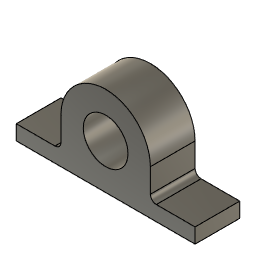
Tutorial Part 3 v1 (Autodesk Fusion 360 design; units mm, degrees)
Autodesk Fusion 360 part; units mm, degrees
sketch "Sketch1" plane through (0, 0, 0) normal (0, 1, 0) x (1, 0, 0)
  line L0 (-60.0453, 0.0038) -> (60.0453, 0.0038)
  line L1 (60.0453, 0.0038) -> (60.0453, -10.0038)
  line L2 (60.0453, -10.0038) -> (-60.0453, -10.0038)
  line L3 (-60.0453, -10.0038) -> (-60.0453, 0.0038)
  line L4 (-60.0453, 0.0038) -> (60.0453, -10.0038) construction
  line L5 (60.0453, 0.0038) -> (-60.0453, -10.0038) construction
  line L6 (-30, -10) -> (30, -10)
  line L7 (30, -10) -> (30, -30)
  line L8 (-30, -30) -> (-30, -10)
  line L9 (-30, -10) -> (30, -30) construction
  line L10 (30, -10) -> (-30, -30) construction
  arc A0 (-30, -30) -> (30, -30) centre (0, -30) ccw
  circle A1 centre (0, -30) radius 15
  line L11 (30, -30) -> (15, -30)
  line L12 (-15, -30) -> (-30, -30)
  point P0 (0, -5)
  point P1 (0, -20)
  dimension "d3" = 60
  dimension "d4" = 20
  constraint horizontal L0
  constraint perpendicular L0 L1
  constraint parallel L1 L3
  constraint coincident L4 P0
  constraint coincident L5 P0
  constraint horizontal L6
  constraint perpendicular L6 L7
  constraint parallel L6 L11
  constraint parallel L7 L8
  constraint coincident L9 P1
  constraint coincident L10 P1
  constraint coincident L8 L10.end
  constraint coincident L10 L8.start
  constraint concentric A0 A1
  constraint coincident A1 L11.end
  constraint coincident A1 L12.start
  constraint collinear L11 L12
  constraint coincident A0.centre L11
  measures "d3" distance of L7.end L8.start
  measures "d4" distance of L6.start L8.start
sketch "Sketch2" plane through (0, 0, 0) normal (0, 1, 0) x (1, 0, 0)
  line L0 (60, 30) -> (-60, 30)
  line L1 (-60, 30) -> (-60, 20)
  line L2 (-60, 20) -> (-30, 20)
  line L3 (-30, 20) -> (-30, 0)
  arc A0 (-30, 0) -> (30, 0) centre (0, 0) ccw
  line L4 (30, 0) -> (30, 20)
  line L5 (30, 20) -> (60, 20)
  line L6 (60, 20) -> (60, 30)
  dimension "d11" = 120
  dimension "d12" = 60
  dimension "d13" = 30
  dimension "d14" = 30
  dimension "d15" = 10
  constraint horizontal L0
  constraint perpendicular L0 L1
  constraint perpendicular L1 L2
  constraint perpendicular L2 L3
  constraint tangent L3 A0
  constraint perpendicular L2 L4
  constraint perpendicular L4 L5
  constraint perpendicular L0 L6
  constraint tangent A0 L4
  constraint coincident A0.centre origin
  constraint collinear L2 L5
  measures "d11" distance of L0.start L0.end
  measures "d12" distance of L1 A0.centre
  measures "d13" radius of A0
  measures "d14" distance of A0.centre L0
  measures "d15" distance of L0.start L5.end
extrude "Extrude2" add sketch "Sketch2" along normal blind 30
sketch "Sketch3" plane through (0, 0, 0) normal (0, -1, 0) x (1, 0, 0)
  line L0 (60, -30) -> (60, -20)
  line L1 (60, -20) -> (30, -20)
  line L2 (30, -20) -> (30, 0)
  arc A0 (30, 0) -> (-30, 0) centre (0, 0) ccw
  line L3 (-30, 0) -> (-30, -20)
  line L4 (-30, -20) -> (-60, -20)
  line L5 (-60, -20) -> (-60, -30)
  line L6 (-60, -30) -> (60, -30)
  circle A1 centre (0, 0) radius 15
  dimension "d18" = 30
  constraint coincident A0.centre A1.centre
  measures "d18" diameter of A1
extrude "Extrude3" cut sketch "Sketch3" against normal blind 30 contours A1
fillet "Fillet5" radius 4 2 edges at (-30, 15, -20) (30, 15, -20)
